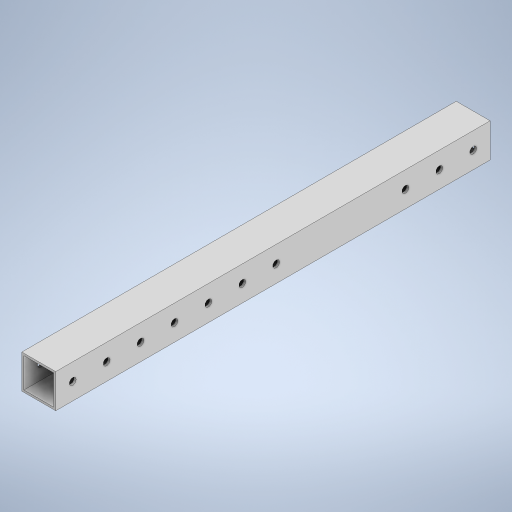
# Autodesk Inventor part: 24in long 1in square tube
Saved by Autodesk Inventor 2024 (Build 280153000, 153)
## iProperties
Created: 2024-01-10
Part Number: 24in long 1in square tube
Material: Generic
Document SubType Name: Modeling
Designer: david
Density: 1 g/cm^3
Appearance: Default
Author: david
Autodesk Inventor part; units mm, degrees
ref_plane "YZ Plane" through (0, 0, 0) normal (1, 0, 0) x (0, 1, 0)
ref_plane "XZ Plane" through (0, 0, 0) normal (0, 1, 0) x (-1, 0, 0)
ref_plane "XY Plane" through (0, 0, 0) normal (0, 0, 1) x (1, 0, 0)
sketch "Sketch1" plane through (0, 0, 0) normal (0, 0, 1) x (1, 0, 0)
  line L0 (-12.7, -12.7) -> (-12.7, 12.7)
  line L1 (-12.7, 12.7) -> (12.7, 12.7)
  line L2 (12.7, 12.7) -> (12.7, -12.7)
  line L3 (12.7, -12.7) -> (-12.7, -12.7)
  line L4 (-12.7, -12.7) -> (12.7, 12.7) construction
  line L5 (-12.7, 12.7) -> (12.7, -12.7) construction
  line L6 (11.1125, 11.1125) -> (-11.1125, 11.1125)
  line L7 (-11.1125, 11.1125) -> (-11.1125, -11.1125)
  line L8 (-11.1125, -11.1125) -> (11.1125, -11.1125)
  line L9 (11.1125, -11.1125) -> (11.1125, 11.1125)
  point P0 (0, 0)
  dimension "d0" = 25.4
  dimension "d1" = 25.4
  dimension "d2" = 1.5875
  constraints: 20 end point, 4 parallel, 2 midpoint, 2 perpendicular, 1 vertical, 3 other
  measures "d0" distance of L0.end L1.end
  measures "d1" distance of L1.end L2.end
  measures "d2" distance between parallel lines of L1 L6
extrude "Extrusion1" add sketch "Sketch1" along normal blind 609.6
sketch "Sketch2" plane through (12.7, -12.7, 0) normal (1, 0, 0) x (0, 0, -1)
  line L0 (0, 0) -> (0, 25.4) projected
  line L1 (0, 25.4) -> (-609.6, 25.4) projected
  line L2 (-609.6, 0) -> (-609.6, 25.4) projected
  line L3 (0, 0) -> (-609.6, 0) projected
  circle A0 centre (-596.9, 12.7) radius 2.5781
  circle A1 centre (-571.5, 12.7) radius 2.5781
  circle A2 centre (-546.1, 12.7) radius 2.5781
  line L4 (-304.8, 0) -> (-304.8, 25.4) construction
  circle A3 centre (-12.7, 12.7) radius 2.5781
  circle A4 centre (-38.1, 12.7) radius 2.5781
  circle A5 centre (-63.5, 12.7) radius 2.5781
  point P0 (0, 12.7)
  dimension "d5" = 5.1562
  dimension "d7" = 12.7
  dimension "d8" = 25.4
  dimension "d9" = 25.4
  constraints: 6 centre point, 3 symmetric about line, 2 end point, 2 midpoint, 1 equal radius, 3 other
  measures "d5" diameter of A0
  measures "d7" distance from line of A0.centre L2
  measures "d8" distance of A1.centre A0.centre
  measures "d9" distance of A2.centre A1.centre
extrude "Extrusion2" cut sketch "Sketch2" against normal through all contours A0 | A1 | A2 | A3 | A4 | A5
sketch "Sketch5" plane through (-12.7, 12.7, 0) normal (0, 1, 0) x (1, 0, 0)
  line L0 (25.4, 0) -> (25.4, -609.6) projected
  line L1 (25.4, 0) -> (25.4, -223.7994)
  line L2 (25.4, -223.7994) -> (-0.9, -223.7994)
  line L3 (-0.9, -223.7994) -> (-0.9, -681.5571)
  line L4 (-0.9, -681.5571) -> (85.6151, -690.7866)
  line L5 (85.6151, -690.7866) -> (25.4, -223.7994)
  point P0 (12.7, 0)
  dimension "d15" = 223.7994
  constraints: 10 end point, 2 perpendicular, 1 point on line
  measures "d15" distance of L0.start L1.end
extrude "Extrusion4" cut sketch "Sketch5" against normal blind 101.6
sketch "Sketch6" plane through (12.7, -12.7, 0) normal (1, 0, 0) x (0, 0, -1)
  line L0 (-223.7994, 1.5875) -> (-223.7994, 23.8125) projected
  line L1 (-223.7994, 12.7) -> (-211.0994, 12.7)
  circle A0 centre (-211.0994, 12.7) radius 2.5781
  line L2 (-211.0994, 12.7) -> (-185.6994, 12.7)
  circle A1 centre (-185.6994, 12.7) radius 2.5781
  line L3 (-185.6994, 12.7) -> (-160.2994, 12.7)
  circle A2 centre (-160.2994, 12.7) radius 2.5781
  point P0 (0, 12.7)
  dimension "d18" = 12.7
  dimension "d19" = 5.1562
  dimension "d20" = 25.4
  dimension "d21" = 5.1562
  dimension "d22" = 25.4
  dimension "d23" = 5.1562
  constraints: 6 end point, 3 centre point, 3 coincident, 3 horizontal, 1 midpoint
  measures "d18" distance of L1.start L1.end
  measures "d19" diameter of A0
  measures "d20" distance of L2.start L2.end
  measures "d21" diameter of A1
  measures "d22" distance of L3.start L3.end
  measures "d23" diameter of A2
extrude "Extrusion5" cut sketch "Sketch6" against normal blind 50.8
sketch "Sketch7" plane through (-12.7, 12.7, 223.7994) normal (0, 0, 1) x (1, 0, 0)
  line L0 (0, -25.4) -> (0, 0) projected
  line L1 (25.4, -25.4) -> (0, -25.4) projected
  line L2 (25.4, 0) -> (25.4, -25.4) projected
  line L3 (0, 0) -> (25.4, 0) projected
  line L4 (23.8125, -1.5875) -> (1.5875, -1.5875) projected
  line L5 (23.8125, -23.8125) -> (23.8125, -1.5875) projected
  line L6 (1.5875, -23.8125) -> (23.8125, -23.8125) projected
  line L7 (1.5875, -1.5875) -> (1.5875, -23.8125) projected
  point P0 (12.7, -12.7)
extrude "Extrusion6" add sketch "Sketch7" along normal blind 127
sketch "Sketch8" plane through (12.7, -12.7, 0) normal (1, 0, 0) x (0, 0, -1)
  circle A0 centre (-211.0994, 12.7) radius 2.5781 projected
  line L0 (-211.0994, 12.7) -> (-236.4994, 12.7)
  line L1 (-236.4994, 12.7) -> (-261.8994, 12.7)
  circle A1 centre (-236.4994, 12.7) radius 2.5781
  circle A2 centre (-261.8994, 12.7) radius 2.5781
  line L2 (-350.7994, 25.4) -> (-350.7994, 0) projected
  line L3 (-350.7994, 12.7) -> (-338.0994, 12.7)
  line L4 (-338.0994, 12.7) -> (-312.6994, 12.7)
  line L5 (-312.6994, 12.7) -> (-287.2994, 12.7)
  circle A3 centre (-287.2994, 12.7) radius 2.5781
  circle A4 centre (-338.0994, 12.7) radius 2.5781
  circle A5 centre (-312.6994, 12.7) radius 2.5781
  point P0 (0, 12.7)
  dimension "d28" = 25.4
  dimension "d29" = 25.4
  dimension "d30" = 5.1562
  dimension "d31" = 5.1562
  dimension "d32" = 12.7
  dimension "d33" = 25.4
  dimension "d34" = 25.4
  dimension "d35" = 5.1562
  dimension "d36" = 5.1562
  dimension "d37" = 5.1562
  constraints: 10 end point, 5 centre point, 5 coincident, 3 point on line, 2 horizontal, 1 midpoint
  measures "d28" distance of L0.start L0.end
  measures "d29" distance of L0.end L1.end
  measures "d30" diameter of A1
  measures "d31" diameter of A2
  measures "d32" distance of L3.start L3.end
  measures "d33" distance of L3.end L4.end
  measures "d34" distance of L4.end L5.end
  measures "d35" diameter of A3
  measures "d36" diameter of A4
  measures "d37" diameter of A5
extrude "Extrusion7" cut sketch "Sketch8" against normal blind 92.075 contours A2 | A1 L1 L0 | L0 L1 A1 | A4 L4 L3 | A3 | A5 L5 L4 | L4 L5 A5 | L3 L4 A4
sketch "Sketch9" plane through (0, 0, 0) normal (0, 0, -1) x (-1, 0, 0)
  line L0 (-12.7, -12.7) -> (-12.7, 12.7) projected
  line L1 (12.7, -12.7) -> (-12.7, -12.7) projected
  line L2 (12.7, 12.7) -> (12.7, -12.7) projected
  line L3 (-12.7, 12.7) -> (12.7, 12.7) projected
  line L4 (-11.1125, 11.1125) -> (-11.1125, -11.1125) projected
  line L5 (11.1125, 11.1125) -> (-11.1125, 11.1125) projected
  line L6 (11.1125, -11.1125) -> (11.1125, 11.1125) projected
  line L7 (-11.1125, -11.1125) -> (11.1125, -11.1125) projected
  point P0 (0, 0)
extrude "Extrusion8" add sketch "Sketch9" along normal blind 152.4
sketch "Sketch10" plane through (12.7, -12.7, 350.7994) normal (1, 0, 0) x (0, 0, -1)
  line L0 (503.1994, 25.4) -> (503.1994, 0) projected
  line L1 (503.1994, 12.7) -> (490.4994, 12.7)
  line L2 (490.4994, 12.7) -> (465.0994, 12.7)
  line L3 (465.0994, 12.7) -> (439.6994, 12.7)
  circle A0 centre (439.6994, 12.7) radius 2.5781
  circle A1 centre (465.0994, 12.7) radius 2.5781
  circle A2 centre (490.4994, 12.7) radius 2.5781
  point P0 (350.7994, 12.7)
  dimension "d42" = 12.7
  dimension "d43" = 25.4
  dimension "d44" = 25.4
  dimension "d45" = 5.1562
  dimension "d46" = 5.1562
  dimension "d47" = 5.1562
  constraints: 6 end point, 3 centre point, 3 coincident, 2 point on line, 1 horizontal, 1 midpoint
  measures "d42" distance of L1.start L1.end
  measures "d43" distance of L1.end L2.end
  measures "d44" distance of L2.end L3.end
  measures "d45" diameter of A0
  measures "d46" diameter of A1
  measures "d47" diameter of A2
extrude "Extrusion9" cut sketch "Sketch10" against normal blind 123.825
sketch "Sketch11" plane through (0, 0, -152.4) normal (0, 0, -1) x (-1, 0, 0)
  line L0 (12.7, -12.7) -> (12.7, 12.7) projected
  line L1 (12.7, 12.7) -> (-12.7, 12.7) projected
  line L2 (-12.7, 12.7) -> (-12.7, -12.7) projected
  line L3 (-12.7, -12.7) -> (12.7, -12.7) projected
  line L4 (-11.1125, 11.1125) -> (11.1125, 11.1125) projected
  line L5 (11.1125, 11.1125) -> (11.1125, -11.1125) projected
  line L6 (11.1125, -11.1125) -> (-11.1125, -11.1125) projected
  line L7 (-11.1125, -11.1125) -> (-11.1125, 11.1125) projected
  point P0 (0, 0)
extrude "Extrusion10" cut sketch "Sketch11" against normal blind 152.4
sketch "Sketch12" plane through (-12.7, 12.7, 350.7994) normal (0, 0, 1) x (1, 0, 0)
  line L0 (25.4, -25.4) -> (25.4, 0) projected
  line L1 (25.4, 0) -> (0, 0) projected
  line L2 (0, 0) -> (0, -25.4) projected
  line L3 (0, -25.4) -> (25.4, -25.4) projected
  line L4 (23.8125, -1.5875) -> (23.8125, -23.8125) projected
  line L5 (23.8125, -23.8125) -> (1.5875, -23.8125) projected
  line L6 (1.5875, -23.8125) -> (1.5875, -1.5875) projected
  line L7 (1.5875, -1.5875) -> (23.8125, -1.5875) projected
  point P0 (12.7, -12.7)
extrude "Extrusion11" add sketch "Sketch12" along normal blind 63.5
sketch "Sketch13" plane through (12.7, -12.7, 0) normal (1, 0, 0) x (0, 0, -1)
  circle A0 centre (-338.0994, 12.7) radius 2.5781 projected
  line L0 (-338.0994, 12.7) -> (-363.4994, 12.7)
  line L1 (-363.4994, 12.7) -> (-388.8994, 12.7)
  line L2 (-388.8994, 12.7) -> (-414.2994, 12.7)
  circle A1 centre (-363.4994, 12.7) radius 2.5781
  circle A2 centre (-388.8994, 12.7) radius 2.5781
  circle A3 centre (-414.2994, 12.7) radius 2.5781
  point P0 (0, 12.7)
  dimension "d54" = 25.4
  dimension "d55" = 25.4
  dimension "d58" = 25.4
  dimension "d59" = 5.1562
  dimension "d60" = 5.1562
  dimension "d61" = 5.1562
  constraints: 6 end point, 3 centre point, 3 coincident, 2 horizontal, 1 point on line
  measures "d54" distance of L0.start L0.end
  measures "d55" distance of L0.end L1.end
  measures "d58" distance of L1.end L2.end
  measures "d59" diameter of A1
  measures "d60" diameter of A2
  measures "d61" diameter of A3
sketch "Sketch14" plane through (-12.7, 12.7, 414.2994) normal (0, 0, 1) x (1, 0, 0)
  line L0 (25.4, 0) -> (0, 0) projected
  line L1 (0, 0) -> (0, -25.4) projected
  line L2 (0, -25.4) -> (25.4, -25.4) projected
  line L3 (25.4, -25.4) -> (25.4, 0) projected
  line L4 (23.8125, -1.5875) -> (23.8125, -23.8125) projected
  line L5 (23.8125, -23.8125) -> (1.5875, -23.8125) projected
  line L6 (1.5875, -23.8125) -> (1.5875, -1.5875) projected
  line L7 (1.5875, -1.5875) -> (23.8125, -1.5875) projected
  point P0 (12.7, -12.7)
extrude "Extrusion12" add sketch "Sketch14" along normal blind 12.7
extrude "Extrusion13" cut sketch "Sketch13" against normal blind 47.625 contours A3 | A2 L2 L1 | L1 L2 A2 | A1 L1 L0 | L0 L1 A1
sketch "Sketch15" plane through (12.7, -12.7, 0) normal (1, 0, 0) x (0, 0, -1)
  circle A0 centre (-363.4994, 12.7) radius 2.5781 projected
  line L0 (-363.4994, 12.7) -> (-376.1994, 12.7)
  line L1 (-376.1994, 12.7) -> (-376.1994, 25.4)
  line L2 (0, 25.4) -> (-426.9994, 25.4) projected
  line L3 (-376.1994, 12.7) -> (-376.1994, -0.0996)
  line L4 (-376.1994, -0.0996) -> (-376.1994, -3.0916)
  line L5 (-376.1994, -3.0916) -> (-480.1709, -3.0916)
  line L6 (-480.1709, -3.0916) -> (-483.3081, 73.6134)
  line L7 (-483.3081, 73.6134) -> (-376.1994, 25.4)
  point P0 (0, 12.7)
  dimension "d64" = 12.7
  constraints: 14 end point, 3 point on line, 2 perpendicular, 1 horizontal
  measures "d64" distance of L0.start L0.end
extrude "Extrusion14" cut sketch "Sketch15" against normal blind 47.625 contours L3 L4 L5 L6 L7 L1
sketch "Sketch17" plane through (12.7, -12.7, 0) normal (1, 0, 0) x (0, 0, -1)
  circle A0 centre (-312.6994, 12.7) radius 2.5781 projected
  line L0 (-312.6994, 12.7) -> (-325.3994, 12.7)
  line L1 (0, 25.4) -> (-376.1994, 25.4) projected
  line L2 (-325.3994, 25.4) -> (-387.8769, 25.4)
  line L3 (-387.8769, 25.4) -> (-387.8769, -7.9808)
  line L4 (-387.8769, -7.9808) -> (-325.3994, -7.9808)
  line L5 (-325.3994, -7.9808) -> (-325.3994, 25.4)
  point P0 (0, 12.7)
  dimension "d67" = 12.7
  constraints: 10 end point, 2 horizontal, 2 parallel, 1 perpendicular, 1 point on line
  measures "d67" distance of L0.start L0.end
extrude "Extrusion15" cut sketch "Sketch17" against normal blind 112.7125 contours L5 L4 L3 L2 L1
equation "\"d1\" = d0"
body "Solid1"
